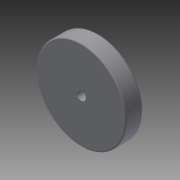
# Autodesk Inventor part: wheel
Saved by Autodesk Inventor 2014 SP1 (Build 180222100, 222)
## iProperties
Created: 2014-09-21
Part Number: wheel
Material: Générique
Document SubType Name: Modeling
Designer: astralien3000
Density: 1 g/cm^3
Appearance: Par défaut
d0: 75,000 mm
d1: 3,000 mm
d2: 0,00 deg
d3: 15,000 mm
d4: 20,000 mm
d5: 12,000 mm
d6: 0,00 deg
d7: 8,000 mm
d9: 0,00 deg
d10: 2,000 mm
d11: 1,000 mm
d12: 1,000 mm
d13: 1,000 mm
d14: 1,000 mm
Author: astralien3000
Autodesk Inventor part; units mm, degrees
ref_plane "YZ Plane" through (0, 0, 0) normal (1, 0, 0) x (0, 1, 0)
ref_plane "XZ Plane" through (0, 0, 0) normal (0, 1, 0) x (-1, 0, 0)
ref_plane "XY Plane" through (0, 0, 0) normal (0, 0, 1) x (1, 0, 0)
sketch "Esquisse1" plane through (0, 0, 0) normal (0, 1, 0) x (-1, 0, 0)
  circle A0 centre (0, 0) radius 37.5
  dimension "d0" = 75
  constraints: 1 centre point, 1 coincident
  measures "d0" diameter of A0
extrude "Extrusion1" add sketch "Esquisse1" along normal blind 3
sketch "Esquisse2" plane through (0, 3, 0) normal (0, 1, 0) x (1, 0, 0)
  circle A0 centre (0, 0) radius 37.5 projected
  circle A1 centre (0, 0) radius 10
  circle A2 centre (0, 0) radius 22.5
  dimension "d3" = 15
  dimension "d4" = 20
  constraints: 2 centre point, 2 coincident
  measures "d3" radial gap between concentric circles of A0 A2
  measures "d4" diameter of A1
extrude "Extrusion2" add sketch "Esquisse2" along normal blind 12
sketch "Esquisse3" plane through (0, 15, 0) normal (0, 1, 0) x (1, 0, 0)
  circle A0 centre (0, 0) radius 10 projected
  circle A1 centre (0, 0) radius 4
  dimension "d7" = 8
  constraints: 1 centre point, 1 coincident
  measures "d7" diameter of A1
extrude "Extrusion3" cut sketch "Esquisse3" against normal through all contours A1
fillet "Congé1" radius 2 1 edges at (-37.5, 15, 0)
fillet "Congé2" radius 1 1 edges at (-10, 15, 0)
fillet "Congé3" radius 1 1 edges at (-22.5, 15, 0)
fillet "Congé4" radius 1 1 edges at (-22.5, 3, 0)
fillet "Congé5" radius 1 1 edges at (37.5, 0, 0)
